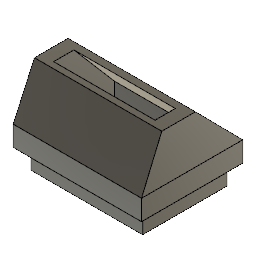
FBG5_fan_duct (Autodesk Fusion 360 design; units mm, degrees)
Autodesk Fusion 360 part; units mm, degrees
sketch "Sketch1" plane through (0, 0, 0) normal (0, 0, 1) x (1, 0, 0)
  line L0 (-8.7725, 5.8867) -> (7.7775, 5.8867)
  line L1 (7.7775, 5.8867) -> (7.7775, -6.6133)
  line L2 (7.7775, -6.6133) -> (-8.7725, -6.6133)
  line L3 (-8.7725, -6.6133) -> (-8.7725, 5.8867)
  line L4 (-8, 5) -> (6.9982, 5)
  line L5 (6.9982, 5) -> (6.9982, -5.595)
  line L6 (6.9982, -5.595) -> (-8, -5.595)
  line L7 (-8, -5.595) -> (-8, 5)
  dimension "d1" = 16.55
  dimension "d2" = 12.5
  constraint horizontal L0
  constraint vertical L1
  constraint horizontal L2
  constraint vertical L3
  constraint horizontal L4
  constraint vertical L5
  constraint horizontal L6
  constraint vertical L7
  measures "d1" distance of L0.start L0.end
  measures "d2" distance of L0.start L2.end
extrude "Extrude1" add sketch "Sketch1" along normal blind 3
sketch "Sketch2" plane through (0, 0, 3) normal (0, 0, 1) x (-1, 0, 0)
  line L0 (-6.9982, 5.595) -> (8, 5.595)
  line L1 (8, 5.595) -> (8, -5)
  line L2 (8, -5) -> (-6.9982, -5)
  line L3 (-6.9982, -5) -> (-6.9982, 5.595)
  line L4 (8.7725, 6.6133) -> (-7.7775, 6.6133)
  line L5 (-7.7775, 6.6133) -> (-7.7775, -5.8867)
  line L6 (-7.7775, -5.8867) -> (8.7725, -5.8867)
  line L7 (8.7725, -5.8867) -> (8.7725, 6.6133)
  line L8 (10, -7) -> (-9, -7)
  line L9 (-9, -7) -> (-9, 8)
  line L10 (-9, 8) -> (10, 8)
  line L11 (10, 8) -> (10, -7)
  constraint horizontal L8
  constraint vertical L9
  constraint horizontal L10
  constraint vertical L11
extrude "Extrude2" add sketch "Sketch2" along normal blind 3 contours L4 L5 L6 L7 | L8 L9 L10 L11
ref_plane "WorkPlane1" through (-0.5, -0.5, 13) normal (0, 0, 1) x (1, 0, 0)
sketch "Sketch4" plane through (-0.5, -0.5, 13) normal (0, 0, 1) x (1, 0, 0)
  line L0 (-9.442, -4.4154) -> (9.4117, -4.4154)
  line L1 (9.4117, -4.4154) -> (9.4117, 0.5846)
  line L2 (9.4117, 0.5846) -> (-9.442, 0.5846)
  line L3 (-9.442, 0.5846) -> (-9.442, -4.4154)
  line L4 (-7.5524, -2.9878) -> (7.4802, -2.9878)
  line L5 (7.4802, -2.9878) -> (7.4802, -0.7203)
  line L6 (7.4802, -0.7203) -> (-7.5524, -0.7203)
  line L7 (-7.5524, -0.7203) -> (-7.5524, -2.9878)
  dimension "d8" = 5
  constraint horizontal L0
  constraint vertical L1
  constraint horizontal L2
  constraint vertical L3
  constraint horizontal L4
  constraint vertical L5
  constraint horizontal L6
  constraint vertical L7
  measures "d8" distance of L0.start L2.end
sketch "Sketch5" plane through (0, 0, 6) normal (0, 0, 1) x (-1, 0, 0)
  line L0 (8, -5) -> (-6.9982, -5)
  line L1 (-6.9982, -5) -> (-6.9982, 5.595)
  line L2 (-6.9982, 5.595) -> (8, 5.595)
  line L3 (8, 5.595) -> (8, -5)
  line L4 (10, 8) -> (-9, 8)
  line L5 (-9, 8) -> (-9, -7)
  line L6 (-9, -7) -> (10, -7)
  line L7 (10, -7) -> (10, 8)
  line L8 (10, -7) -> (-9, -7)
  line L9 (-9, -7) -> (-9, 8)
  line L10 (-9, 8) -> (10, 8)
  line L11 (10, 8) -> (10, -7)
  constraint horizontal L8
  constraint vertical L9
  constraint horizontal L10
  constraint vertical L11
  constraint coincident L4.end L5.start
  constraint coincident L6.end L7.start
loft "Loft1" add profiles "Sketch5", "Sketch4" section 1 section 2
sketch "Sketch6" plane through (0, 0, 13) normal (0, 0, 1) x (-1, 0, 0)
  line L0 (9.942, 4.9154) -> (-8.9117, 4.9154)
  line L1 (-8.9117, 4.9154) -> (-8.9117, -0.0846)
  line L2 (-8.9117, -0.0846) -> (9.942, -0.0846)
  line L3 (9.942, -0.0846) -> (9.942, 4.9154)
  line L4 (8, 1) -> (-7, 1)
  line L5 (-7, 1) -> (-7, 4)
  line L6 (-7, 4) -> (8, 4)
  line L7 (8, 4) -> (8, 1)
  constraint horizontal L4
  constraint vertical L5
  constraint horizontal L6
  constraint vertical L7
sketch "Sketch7" plane through (0, 0, 6) normal (0, 0, -1) x (1, 0, 0)
  line L0 (6.9982, -5) -> (6.9982, 5.595)
  line L1 (6.9982, 5.595) -> (-8, 5.595)
  line L2 (-8, 5.595) -> (-8, -5)
  line L3 (-8, -5) -> (6.9982, -5)
  line L4 (-8, 5.595) -> (6.9982, 5.595)
  line L5 (6.9982, 5.595) -> (6.9982, -5)
  line L6 (6.9982, -5) -> (-8, -5)
  line L7 (-8, -5) -> (-8, 5.595)
  constraint horizontal L4
  constraint vertical L5
  constraint horizontal L6
  constraint vertical L7
  constraint coincident L0.start L3.end
  constraint coincident L1.end L2.start
loft "Loft2" cut profiles "Sketch7", "Sketch6" section 1 section 2 contours L4 L5 L6 L7
